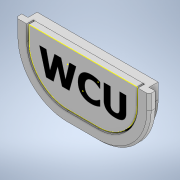
# Autodesk Inventor part: LOGO_Holder_inside
Saved by Autodesk Inventor 2022 (Build 260153000, 153)
## iProperties
Created: 2021-04-23
Part Number: LOGO_Holder_inside
Material: Generic
Document SubType Name: Modeling
Designer: Viktor
Density: 1 g/cm^3
Appearance: Default
Author: Viktor
## iProperties of the stored document LOGO_Holder_inside_3DPrint.ipt
Created: 2021-04-23
Part Number: LOGO_Holder_inside_3DPrint
Material: Generic
Document SubType Name: Modeling
Designer: Viktor
Density: 1 g/cm^3
Appearance: Default
Author: Viktor
Autodesk Inventor part; units mm, degrees
ref_plane "YZ Plane" through (0, 0, 0) normal (1, 0, 0) x (0, 1, 0)
ref_plane "XZ Plane" through (0, 0, 0) normal (0, 1, 0) x (-1, 0, 0)
ref_plane "XY Plane" through (0, 0, 0) normal (0, 0, 1) x (1, 0, 0)
sketch "Sketch1" plane through (0, 0, 0) normal (0, 0, 1) x (1, 0, 0)
  line L0 (-20, -10) -> (20, -10)
  line L1 (20, -10) -> (20, 10)
  line L2 (20, 10) -> (-20, 10)
  line L3 (-20, 10) -> (-20, -10)
  line L4 (-20, -10) -> (20, 10) construction
  line L5 (20, -10) -> (-20, 10) construction
  point P0 (0, 0)
  dimension "d0" = 40
  dimension "d1" = 20
  constraints: 12 end point, 2 midpoint, 2 parallel, 1 horizontal, 1 perpendicular
  measures "d0" distance of L1.end L2.end
  measures "d1" distance of L0.end L1.end
extrude "Extrusion1" add sketch "Sketch1" along normal blind 5
fillet "Fillet1" radius 15 2 edges at (20, -10, 2.5) (-20, -10, 2.5)
thicken "Thicken1" operation add thickness 0.2 both sides no extend neighbours yes toward (-1, 0, 0) faces at (20, 6.6667, 3.3333) (19.9581, 3.879, 1.6667) (-1.6667, -10, 1.6667) (-7.2356, -9.8325, 1.6667) (-20, 8.3333, 1.6667)
sketch "Sketch2" plane through (0, 0, 5) normal (0, 0, 1) x (1, 0, 0)
  line L0 (-19.8, 10) -> (-19.8, 5) projected
  arc A0 (-19.8, 5) -> (-5, -9.8) centre (-5, 5) ccw projected
  line L1 (-5, -9.8) -> (5, -9.8) projected
  arc A1 (5, -9.8) -> (19.8, 5) centre (5, 5) ccw projected
  line L2 (19.8, 5) -> (19.8, 10) projected
  line L3 (-21.8, 10) -> (-21.8, 5)
  arc A2 (-21.8, 5) -> (-5, -11.8) centre (-5, 5) ccw
  line L4 (-5, -11.8) -> (5, -11.8)
  arc A3 (5, -11.8) -> (21.8, 5) centre (5, 5) ccw
  line L5 (21.8, 5) -> (21.8, 10)
  line L6 (-21.8, 10) -> (21.8, 10)
  point P0 (0, 0)
  dimension "d7" = 2
  constraints: 8 end point, 4 point on circle, 2 centre point, 2 point on line, 4 other
  measures "d7" distance between parallel lines of L0 L3
extrude "Extrusion2" add sketch "Sketch2" against normal blind 2 contours L0 A0 L1 A1 L2 L6 L5 A3 L4 A2 L3
chamfer "Chamfer1" distance 0.7 angle 45 5 edges at (-16.8794, -6.8794, 5) (0, -11.8, 5) (16.8794, -6.8794, 5) (21.8, 7.5, 5) (-21.8, 7.5, 5)
sketch "Sketch3" plane through (0, 0, 5) normal (0, 0, 1) x (1, 0, 0)
  arc A0 (-19.8, 5) -> (-5, -9.8) centre (-5, 5) ccw projected
  line L0 (-19.8, 10) -> (-19.8, 5) projected
  line L1 (-5, -9.8) -> (5, -9.8) projected
  arc A1 (5, -9.8) -> (19.8, 5) centre (5, 5) ccw projected
  line L2 (19.8, 5) -> (19.8, 10) projected
  line L3 (-18.2, 10) -> (-18.2, 5)
  arc A2 (-18.2, 5) -> (-5, -8.2) centre (-5, 5) ccw
  line L4 (-5, -8.2) -> (5, -8.2)
  arc A3 (5, -8.2) -> (18.2, 5) centre (5, 5) ccw
  line L5 (18.2, 5) -> (18.2, 10)
  line L6 (21.1, 10) -> (-21.1, 10) projected
  point P0 (0, 0)
  dimension "d13" = 1.6
  constraints: 6 end point, 4 point on circle, 2 centre point, 4 other
  measures "d13" distance between parallel lines of L0 L3
extrude "Extrusion3" cut sketch "Sketch3" against normal blind 2.2 contours L6 L5 A3 L4 A2 L3
sketch "Sketch4" plane through (0, 0, 2.8) normal (0, 0, 1) x (1, 0, 0)
  line L0 (-18.2, 5) -> (-18.2, 10) projected
  arc A0 (-18.2, 5) -> (-5, -8.2) centre (-5, 5) ccw projected
  line L1 (5, -8.2) -> (-5, -8.2) projected
  arc A1 (5, -8.2) -> (18.2, 5) centre (5, 5) ccw projected
  line L2 (18.2, 10) -> (18.2, 5) projected
  line L3 (-17.7, 10) -> (-17.7, 5)
  arc A2 (-17.7, 5) -> (-5, -7.7) centre (-5, 5) ccw
  line L4 (-5, -7.7) -> (5, -7.7)
  arc A3 (5, -7.7) -> (17.7, 5) centre (5, 5) ccw
  line L5 (17.7, 5) -> (17.7, 10)
  line L6 (-18.2, 10) -> (18.2, 10) projected
  point P0 (0, 0)
  dimension "d16" = 0.5
  constraints: 6 end point, 4 point on circle, 2 centre point, 4 other
  measures "d16" distance between parallel lines of L0 L3
extrude "Extrusion4" add sketch "Sketch4" along normal blind 2 separate body contours L6 L5 A3 L4 A2 L3
sketch "Sketch5" plane through (0, 0, 4.8) normal (0, 0, 1) x (1, 0, 0)
  line L0 (-14.4662, 5.9663) -> (5.9545, 5.9663) construction
  line L1 (5.9545, 5.9663) -> (5.9545, -0.3809) construction
  line L2 (5.9545, -0.3809) -> (-14.4662, -0.3809) construction
  line L3 (-14.4662, -0.3809) -> (-14.4662, 5.9663) construction
  line L4 (17.7, 5) -> (17.7, 10) projected
  line L5 (17.7, 10) -> (-17.7, 10) projected
  line L6 (-17.7, 10) -> (-17.7, 5) projected
  arc A0 (-17.7, 5) -> (-5, -7.7) centre (-5, 5) ccw projected
  line L7 (-5, -7.7) -> (5, -7.7) projected
  arc A1 (5, -7.7) -> (17.7, 5) centre (5, 5) ccw projected
  point P0 (0, 0)
  constraints: 2 other
body "Solid1"
body "Solid2"
